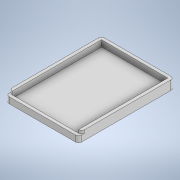
# Autodesk Inventor part: esp_shield_holder
Saved by Autodesk Inventor 2021 (Build 250183000, 183)
## iProperties
Created: 2024-05-20
Part Number: esp_shield_holder
Material: Generic
Document SubType Name: Modeling
Designer: 23adrdam
Density: 1 g/cm^3
Appearance: Default
Author: 23adrdam
Autodesk Inventor part; units mm, degrees
ref_plane "YZ Plane" through (0, 0, 0) normal (1, 0, 0) x (0, 1, 0)
ref_plane "XZ Plane" through (0, 0, 0) normal (0, 1, 0) x (-1, 0, 0)
ref_plane "XY Plane" through (0, 0, 0) normal (0, 0, 1) x (1, 0, 0)
sketch "Sketch1" plane through (0, 0, 0) normal (0, 1, 0) x (-1, 0, 0)
  line L0 (-23.55, -31) -> (23.55, -31)
  line L1 (23.55, -31) -> (23.55, 31)
  line L2 (23.55, 31) -> (-23.55, 31)
  line L3 (-23.55, 31) -> (-23.55, -31)
  line L4 (-23.55, -31) -> (23.55, 31) construction
  line L5 (23.55, -31) -> (-23.55, 31) construction
  point P0 (0, 0)
  dimension "d0" = 47.1
  dimension "d1" = 62
  constraints: 12 end point, 2 midpoint, 2 parallel, 1 horizontal, 1 perpendicular
  measures "d0" distance of L1.end L2.end
  measures "d1" distance of L0.end L1.end
extrude "Extrusion1" add sketch "Sketch1" along normal blind 2
sketch "Sketch2" plane through (0, 2, 0) normal (0, 1, 0) x (1, 0, 0)
  line L0 (-23.55, 31) -> (-23.55, -31) projected
  line L1 (23.55, -31) -> (23.55, 31) projected
  line L2 (-23.55, -31) -> (23.55, -31)
  line L3 (23.55, -31) -> (23.55, 31)
  line L4 (23.55, 31) -> (-23.55, 31)
  line L5 (-23.55, 31) -> (-23.55, -31)
  line L6 (-21.55, -29) -> (21.55, -29)
  line L7 (21.55, -29) -> (21.55, 29)
  line L8 (21.55, 29) -> (-21.55, 29)
  line L9 (-21.55, 29) -> (-21.55, -29)
  point P0 (0, 0)
  dimension "d4" = 2
  dimension "d5" = 2
  dimension "d6" = 2
  dimension "d7" = 2
  constraints: 16 end point, 4 parallel, 2 horizontal, 2 perpendicular
  measures "d4" distance between parallel lines of L6 L2
  measures "d5" distance between parallel lines of L4 L8
  measures "d6" distance between parallel lines of L1 L7
  measures "d7" distance between parallel lines of L0 L9
extrude "Extrusion2" add sketch "Sketch2" along normal blind 2
sketch "Sketch3" plane through (0, 4, 0) normal (0, 1, 0) x (1, 0, 0)
  line L0 (-23.55, 31) -> (-23.55, -31) projected
  line L1 (23.55, 31) -> (-23.55, 31)
  line L2 (-23.55, 31) -> (-23.55, -29)
  line L3 (23.55, -29) -> (23.55, 31)
  line L4 (21.55, 29) -> (21.55, -29) projected
  line L5 (-21.55, -29) -> (-21.55, 29) projected
  line L6 (21.55, 29) -> (-21.55, 29)
  line L7 (-21.55, 29) -> (-21.55, -29)
  line L8 (-21.55, -29) -> (21.55, -29)
  line L9 (21.55, -29) -> (21.55, 29)
  line L10 (-21.55, -29) -> (-23.55, -29)
  line L11 (21.55, -29) -> (23.55, -29)
  line L12 (23.55, -31) -> (23.55, 31) projected
  line L13 (-23.55, -31) -> (23.55, -31) projected
  point P0 (0, 0)
  constraints: 18 end point, 3 parallel, 3 perpendicular, 2 horizontal, 2 point on line
extrude "Extrusion3" add sketch "Sketch3" along normal blind 2 contours L1 L3 L11 L4 L6 L5 L10 L0
fillet "Fillet1" radius 2 6 edges at (23.55, 2, 31) (23.55, 3, -31) (-23.55, 3, -31) (-23.55, 5, 29) (23.55, 5, 29) (-23.55, 2, 31)
body "Solid1"
